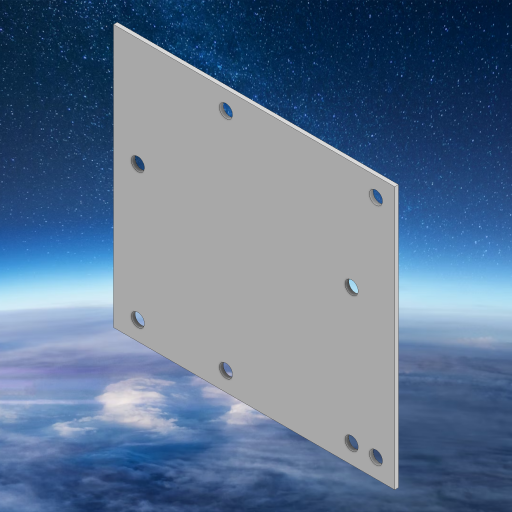
# Autodesk Inventor part: signal_combiner_plate
Saved by Autodesk Inventor 2023 (Build 270158000, 158)
## iProperties
Created: 2023-05-29
Part Number: signal_combiner_plate
Material: 一般
Document SubType Name: Sheet Metal
Designer: 310611102
Density: 1 g/cm^3
Sheet Metal Rule: Default_mm
Appearance: 預設
Author: 310611102
Autodesk Inventor part; units mm, degrees
ref_plane "YZ Plane" through (0, 0, 0) normal (1, 0, 0) x (0, 1, 0)
ref_plane "XZ Plane" through (0, 0, 0) normal (0, 1, 0) x (-1, 0, 0)
ref_plane "XY Plane" through (0, 0, 0) normal (0, 0, 1) x (1, 0, 0)
sketch "Sketch1" plane through (0, 0, 0) normal (0, 0, 1) x (1, 0, 0)
  line L0 (-25, 35) -> (25, 35)
  line L1 (25, 35) -> (25, -35)
  line L2 (25, -35) -> (-25, -35)
  line L3 (-25, -35) -> (-25, 35)
  line L4 (-25, 35) -> (25, -35) construction
  line L5 (25, 35) -> (-25, -35) construction
  circle A0 centre (-20, 30) radius 1.75
  line L6 (0, 0) -> (0, 8.6163)
  line L7 (0, 0) -> (3.549, 0)
  circle A1 centre (20, 30) radius 1.75
  circle A2 centre (-20, -30) radius 1.75
  circle A3 centre (20, -30) radius 1.75
  line L8 (-50, 35) -> (-25, 35)
  line L9 (-25, 35) -> (-25, -35)
  line L10 (-25, -35) -> (-50, -35)
  line L11 (-50, -35) -> (-50, 35)
  line L12 (-50, 35) -> (-25, -35) construction
  line L13 (-25, 35) -> (-50, -35) construction
  point P0 (-37.5, 0)
  point P1 (25, 25)
  dimension "d0" = 50
  dimension "d1" = 70
  dimension "d12" = 3.5
  dimension "d13" = 5
  dimension "d18" = 5
  dimension "d26" = 70
  dimension "d29" = 50
  measures "d0" distance of L0.start L0.end
  measures "d1" distance of L0.end L1.end
  measures "d12" diameter of A0
  measures "d13" distance from line of L0 A0.centre
  measures "d18" distance from line of L3 A0.centre
  measures "d26" distance of L10.end L8.start
  measures "d29" distance from line of L6.start L11
extrude "Plate1" add sketch "Sketch1" along normal blind 1
sketch "Sketch3" plane through (0, 0, 1) normal (0, 0, 1) x (1, 0, 0)
  line L0 (-43.5, 6) -> (13.5, 6) construction
  line L1 (13.5, 6) -> (13.5, -30) construction
  line L2 (13.5, -30) -> (-43.5, -30) construction
  line L3 (-43.5, -30) -> (-43.5, 6) construction
  line L4 (-43.5, 6) -> (13.5, -30) construction
  line L5 (13.5, 6) -> (-43.5, -30) construction
  circle A0 centre (-43.5, 6) radius 1.75
  circle A1 centre (13.5, 6) radius 1.75
  circle A2 centre (13.5, -30) radius 1.75
  circle A3 centre (-43.5, -30) radius 1.75
  point P0 (-15, -12)
  point P1 (0, 0)
  dimension "d22" = 57
  dimension "d23" = 36
  dimension "d24" = 3.5
  dimension "d30" = 15
  dimension "d32" = 30
  constraints: 12 end point, 4 centre point, 4 coincident, 3 equal radius, 2 midpoint, 2 parallel, 1 horizontal, 1 perpendicular
  measures "d22" distance between parallel lines of L1 L3
  measures "d23" distance of L0.end L1.end
  measures "d24" diameter of A0
  measures "d30" horizontal distance of point (0, 0) point (-15, -12)
  measures "d32" vertical distance of point (0, 0) L2.end
extrude "Cut1" cut sketch "Sketch3" against normal blind 1
equation "\"d27\" = 厚度"
equation "\"d2\" = 厚度"
equation "\"折彎半徑\" = 厚度"
equation "\"折彎離隙寬度\" = 厚度"
equation "\"折彎離隙深度\" = 0.5 * 厚度"
equation "\"轉角離隙大小\" = 4 * 厚度"
equation "\"最小剩餘\" = 2 * 厚度"
equation "\"轉移半徑\" = 折彎半徑"
equation "\"Jacobi半徑大小\" = 折彎半徑"
equation "\"間隙大小\" = 厚度"
equation "\"厚度\" = 1"
body "Solid1"
